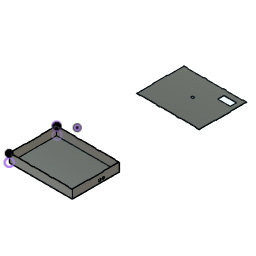
Final Submission (Autodesk Fusion 360 design; units mm, degrees)
Autodesk Fusion 360 part; units mm, degrees
sketch "Sketch1" plane through (0, 0, 0) normal (0, 0, 1) x (1, 0, 0)
  line L0 (-21.9872, 0) -> (-21.9872, 50)
  line L1 (-21.9872, 50) -> (-24.9872, 50)
  line L2 (-21.9872, 50) -> (-21.9872, 40)
  line L3 (-21.9872, 40) -> (-24.9872, 40)
  line L4 (-22, 40) -> (-22, 10)
  line L5 (-22, 10) -> (-25, 10)
  measures "d58" distance of L0.end
box "BoxPrimitive1" add length 300 width 450 height 50 placed x (0, 1, 0) y (-1, 0, 0) z (0, 0, 1) at (450, 0, 0) makes body 1
delete_face "DeleteFace1" 6 faces at (150, 100, 50) (0, 200, 16.6667) (300, 300, 16.6667) (450, 200, 16.6667) (300, 0, 16.6667) (150, 100, 0) on bodies 1
sketch "Sketch2" plane through (0, 0, 0) normal (0, 0, 1) x (1, 0, 0)
sketch "Sketch3" plane through (0, 0, 0) normal (0, 0, 1) x (1, 0, 0)
sketch "Sketch4" plane through (0, 0, 0) normal (0, 0, 1) x (1, 0, 0)
  line L0 (0, 0) -> (400, 0)
  line L1 (400, 0) -> (400, 3)
  line L2 (400, 3) -> (0, 3)
  line L3 (0, 3) -> (0, 0)
  dimension "d8" = 400
  constraint horizontal L0
  constraint vertical L1
  constraint horizontal L2
  constraint vertical L3
  constraint coincident L0.start L3.end
  measures "d8" distance of L0.start L0.end
extrude "Extrude1" add sketch "Sketch4" along normal blind 50 separate body makes body 2
sketch "Sketch5" plane through (0, 0, 0) normal (-1, 0, 0) x (0, -1, 0)
  line L0 (-3, 0) -> (0, 0)
  line L1 (0, 0) -> (0, 50)
  line L2 (0, 50) -> (-3, 50)
  line L3 (-3, 50) -> (-3, 0)
  line L4 (-3, 50) -> (0, 50)
  line L5 (0, 50) -> (0, 40)
  line L6 (0, 40) -> (-3, 40)
  line L7 (-3, 40) -> (-3, 50)
  dimension "d11" = 10
  constraint horizontal L4
  constraint vertical L5
  constraint horizontal L6
  constraint vertical L7
  constraint coincident L2.end L3.start
  measures "d11" distance of L2.end L6.end
sketch "Sketch6" plane through (0, 0, 0) normal (-1, 0, 0) x (0, -1, 0)
extrude "Extrude2" cut sketch "Sketch5" against normal blind 3 contours L1 L2 L3 L4 L5 L6 L7 bodies 2
sketch "Sketch7" plane through (0, 0, 0) normal (-1, 0, 0) x (0, -1, 0)
  line L0 (0, 40) -> (-3, 40)
  line L1 (-3, 40) -> (-3, 0)
  line L2 (-3, 0) -> (0, 0)
  line L3 (0, 0) -> (0, 40)
  line L4 (-3, 10) -> (0, 10)
  line L5 (0, 10) -> (0, 0)
  line L6 (0, 0) -> (-3, 0)
  line L7 (-3, 0) -> (-3, 10)
  constraint horizontal L4
  constraint vertical L5
  constraint horizontal L6
  constraint vertical L7
  constraint coincident L2.end L3.start
  constraint coincident L1 L4.start
extrude "Extrude3" cut sketch "Sketch7" against normal blind 3 contours L1 L2 L3 L4 L5 L6 L7 bodies 2
sketch "Sketch8" plane through (400, 0, 0) normal (1, 0, 0) x (0, 1, 0)
  line L0 (0, 0) -> (3, 0)
  line L1 (3, 0) -> (3, 50)
  line L2 (3, 50) -> (0, 50)
  line L3 (0, 50) -> (0, 0)
  line L4 (0, 50) -> (3.2755, 50)
  line L5 (3.2755, 50) -> (3.2755, 40)
  line L6 (3.2755, 40) -> (0, 40)
  line L7 (0, 40) -> (0, 50)
  line L8 (0, 40) -> (3, 40)
  line L9 (3, 40) -> (3, 10)
  line L10 (3, 10) -> (0, 10)
  line L11 (0, 10) -> (0, 40)
  line L12 (0, 10) -> (3, 10)
  line L13 (3, 10) -> (3, 0)
  line L14 (3, 0) -> (0, 0)
  line L15 (0, 0) -> (0, 10)
  dimension "d17" = 10
  dimension "d18" = 30
  constraint horizontal L4
  constraint vertical L5
  constraint horizontal L6
  constraint vertical L7
  constraint coincident L2.end L3.start
  constraint horizontal L8
  constraint vertical L9
  constraint horizontal L10
  constraint vertical L11
  constraint horizontal L12
  constraint vertical L13
  constraint horizontal L14
  constraint vertical L15
  constraint coincident L0.end L1.start
  measures "d17" distance of L2.end L6.end
  measures "d18" distance of L6.end L10.end
extrude "Extrude4" cut sketch "Sketch8" against normal blind 3 contours L1 L2 L3 L4 L6 L7 L8 bodies 2
sketch "Sketch9" plane through (0, 0, 0) normal (-1, 0, 0) x (0, -1, 0)
sketch "Sketch10" plane through (400, 0, 0) normal (1, 0, 0) x (0, 1, 0)
  line L0 (3, 40) -> (0, 40)
  line L1 (0, 40) -> (0, 0)
  line L2 (0, 0) -> (3, 0)
  line L3 (3, 0) -> (3, 40)
  line L4 (0, 0) -> (3, 0)
  line L5 (3, 0) -> (3, 10)
  line L6 (3, 10) -> (0, 10)
  line L7 (0, 10) -> (0, 0)
  dimension "d23" = 10
  constraint horizontal L4
  constraint vertical L5
  constraint horizontal L6
  constraint vertical L7
  constraint coincident L1.end L2.start
  measures "d23" distance of L1.end L6.end
extrude "Extrude5" cut sketch "Sketch10" against normal blind 3 contours L1 L2 L3 L4 L5 L6 L7 bodies 2
sketch "Sketch13" plane through (0, 0, 0) normal (0, 0, -1) x (1, 0, 0)
sketch "Sketch14" plane through (0, 0, 0) normal (0, 0, -1) x (1, 0, 0)
  line L0 (397, -3) -> (397, 0)
  line L1 (397, 0) -> (3, 0)
  line L2 (3, 0) -> (3, -3)
  line L3 (3, -3) -> (397, -3)
  line L4 (26.5, 0) -> (126.5, 0)
  line L5 (126.5, 0) -> (126.5, -2.9142)
  line L6 (126.5, -2.9142) -> (26.5, -2.9142)
  line L7 (26.5, -2.9142) -> (26.5, 0)
  dimension "d30" = 100
  constraint horizontal L4
  constraint vertical L5
  constraint horizontal L6
  constraint vertical L7
  constraint coincident L1 L4.start
  measures "d30" distance of L4.start L4.end
extrude "Extrude6" add sketch "Sketch14" along normal blind 3 contours L1 L4 L5 L6 L7 bodies 2
sketch "Sketch15" plane through (0, 0, 0) normal (0, 0, -1) x (1, 0, 0)
sketch "Sketch16" plane through (0, 0, 0) normal (0, 0, -1) x (1, 0, 0)
sketch "Sketch17" plane through (0, 0, 0) normal (0, 0, -1) x (1, 0, 0)
  line L0 (150, 0) -> (250, 0)
  line L1 (250, 0) -> (250, -3.0762)
  line L2 (250, -3.0762) -> (150, -3.0762)
  line L3 (150, -3.0762) -> (150, 0)
  dimension "d35" = 100
  constraint horizontal L0
  constraint vertical L1
  constraint horizontal L2
  constraint vertical L3
  measures "d35" distance of L0.start L0.end
sketch "Sketch18" plane through (0, 0, 0) normal (0, 0, -1) x (1, 0, 0)
extrude "Extrude7" add sketch "Sketch17" along normal blind 3 bodies 2
sketch "Sketch19" plane through (0, 0, 0) normal (0, 0, -1) x (1, 0, 0)
sketch "Sketch20" plane through (0, 0, 0) normal (0, 0, -1) x (1, 0, 0)
sketch "Sketch21" plane through (0, 0, 0) normal (0, 0, -1) x (1, 0, 0)
  line L0 (273.5, 0) -> (373.5, 0)
  line L1 (373.5, 0) -> (373.5, -3)
  line L2 (373.5, -3) -> (273.5, -3)
  line L3 (273.5, -3) -> (273.5, 0)
  dimension "d43" = 100
  constraint horizontal L0
  constraint vertical L1
  constraint horizontal L2
  constraint vertical L3
  measures "d43" distance of L0.start L0.end
extrude "Extrude8" add sketch "Sketch21" along normal blind 3 bodies 2
sketch "Sketch23" plane through (0, 0, 0) normal (0, 0, 1) x (1, 0, 0)
sketch "Sketch24" plane through (0, 0, 0) normal (0, 0, 1) x (1, 0, 0)
  line L0 (0, -2) -> (3, -2)
  line L1 (3, -2) -> (3, -302)
  line L2 (3, -302) -> (0, -302)
  line L3 (0, -302) -> (0, -2)
  dimension "d47" = 3
  dimension "d48" = 300
  constraint horizontal L0
  constraint vertical L1
  constraint horizontal L2
  constraint vertical L3
  measures "d47" distance of L0.start L0.end
  measures "d48" distance of L0.start L2.end
sketch "Sketch22" plane through (0, 0, 0) normal (0, -1, 0) x (1, 0, 0)
extrude "Extrude9" add sketch "Sketch24" along normal blind 50 separate body makes body 3
move_body "MoveFace1" bodies 3 to x (1, 0, 0) y (0, 1, 0) z (0, 0, 1) at (-24.9872, -104.133, 0) on bodies 3
sketch "Sketch55" plane through (0, 0, 3) normal (0, 0, 1) x (-1, 0, 0)
  line L0 (-192.7778, -526.1003) -> (-207.7778, -526.1003)
  line L1 (-207.7778, -526.1003) -> (-207.7778, -514.1003)
  line L2 (-207.7778, -514.1003) -> (-192.7778, -514.1003)
  line L3 (-192.7778, -514.1003) -> (-192.7778, -526.1003)
  dimension "d161" = 15
  dimension "d162" = 12
  constraint horizontal L0
  constraint vertical L1
  constraint horizontal L2
  constraint vertical L3
  measures "d161" distance of L0.start L0.end
  measures "d162" distance of L0.start L2.end
sketch "Sketch25" plane through (0, -106.133, 0) normal (0, 1, 0) x (-1, 0, 0)
  line L0 (24.9872, 50) -> (21.9872, 50)
  line L1 (21.9872, 50) -> (24.9872, 50)
  line L2 (21.9872, 40) -> (21.9872, 50)
  dimension "d51" = 10
  constraint horizontal L1
  constraint vertical L2
  constraint coincident L0.end L1.start
  measures "d51" distance of L0.end L2.start
sketch "Sketch56" plane through (0, 0, 3) normal (0, 0, 1) x (1, 0, 0)
sketch "Sketch26" plane through (0, -106.133, 0) normal (0, 1, 0) x (-1, 0, 0)
sketch "Sketch27" plane through (0, -106.133, 0) normal (0, 1, 0) x (-1, 0, 0)
  line L0 (22, 40) -> (25.1085, 40)
  line L1 (25.1085, 40) -> (25.1085, 10)
  line L2 (25.1085, 10) -> (22, 10)
  line L3 (22, 10) -> (22, 40)
  dimension "d54" = 30
  constraint horizontal L0
  constraint vertical L1
  constraint horizontal L2
  constraint vertical L3
  measures "d54" distance of L0.start L2.end
sketch "Sketch28" plane through (0, -106.133, 0) normal (0, 1, 0) x (-1, 0, 0)
extrude "Extrude10" cut sketch "Sketch27" against normal blind 3 bodies 3
delete_face "DeleteFace2" 1 faces at (-22, -108.133, 20) on bodies 3
sketch "Sketch29" plane through (0, -406.133, 0) normal (0, -1, 0) x (1, 0, 0)
  line L0 (-24.9872, 0) -> (-21.9872, 0)
  line L1 (-21.9872, 0) -> (-21.9872, 50)
  line L2 (-21.9872, 50) -> (-24.9872, 50)
  line L3 (-24.9872, 50) -> (-21.9872, 50)
  line L4 (-21.9872, 50) -> (-21.9872, 40)
  line L5 (-21.9872, 40) -> (-24.9872, 40)
  line L6 (-24.9872, 40) -> (-24.9872, 50)
  dimension "d57" = 10
  dimension "d58" = 3
  constraint horizontal L3
  constraint vertical L4
  constraint horizontal L5
  constraint vertical L6
  constraint coincident L2.end L3.start
  measures "d57" distance of L2.end L5.end
  measures "d58" distance of L2.end L1.end
sketch "Sketch30" plane through (0, -406.133, 0) normal (0, -1, 0) x (1, 0, 0)
sketch "Sketch31" plane through (-23.4872, -406.133, 20) normal (0, -1, 0) x (1, 0, 0)
sketch "Sketch32" plane through (-23.4872, -406.133, 20) normal (0, -1, 0) x (1, 0, 0)
sketch "Sketch33" plane through (0, -406.133, 0) normal (0, -1, 0) x (1, 0, 0)
  line L0 (-25, 40) -> (-22, 40)
  line L1 (-22, 40) -> (-22, 10)
  line L2 (-22, 10) -> (-25, 10)
  line L3 (-25, 10) -> (-25, 40)
  constraint horizontal L0
  constraint vertical L1
  constraint horizontal L2
  constraint vertical L3
extrude "Extrude11" cut sketch "Sketch33" against normal blind 3 bodies 3
delete_face "DeleteFace3" 1 faces at (-22, -405.133, 30) on bodies 3
sketch "Sketch34" plane through (0, 0, 0) normal (0, 0, -1) x (1, 0, 0)
  line L0 (-21.9872, 406.133) -> (-24.9872, 406.133)
  line L1 (-21.9872, 106.133) -> (-21.9872, 406.133)
sketch "Sketch35" plane through (0, 0, 0) normal (0, 0, -1) x (1, 0, 0)
  line L0 (-25, 109) -> (-22, 109)
  line L1 (-22, 109) -> (-22, 209)
  line L2 (-22, 209) -> (-25, 209)
  line L3 (-25, 209) -> (-25, 109)
  dimension "d65" = 100
  constraint horizontal L0
  constraint vertical L1
  constraint horizontal L2
  constraint vertical L3
  measures "d65" distance of L0.start L2.end
extrude "Extrude12" add sketch "Sketch35" along normal blind 3 bodies 3
sketch "Sketch36" plane through (0, 0, 0) normal (0, 0, -1) x (1, 0, 0)
sketch "Sketch37" plane through (0, 0, 0) normal (0, 0, -1) x (1, 0, 0)
  line L0 (-25, 403) -> (-22, 403)
  line L1 (-22, 403) -> (-22, 303)
  line L2 (-22, 303) -> (-25, 303)
  line L3 (-25, 303) -> (-25, 403)
  dimension "d69" = 100
  constraint horizontal L0
  constraint vertical L1
  constraint horizontal L2
  constraint vertical L3
  measures "d69" distance of L0.start L2.end
extrude "Extrude13" add sketch "Sketch37" along normal blind 3 bodies 3
copy_body "CopyPasteBodies1" bodies 3 makes body 4
move_body "Move1" bodies 4 to x (1, 0, 0) y (0, 1, 0) z (0, 0, 1) at (550, 0, 0)
copy_body "CopyPasteBodies2" bodies 2 makes body 5
move_body "Move2" bodies 5 to x (1, 0, 0) y (0, 1, 0) z (0, 0, 1) at (0, -430, 0)
move_body "Align1" bodies 5 to x (1, 0, 0) y (0, 1, 0) z (0, 0, 1) at (-24.9872, 23.867, 0)
move_body "Align2" bodies 2 to x (1, 0, 0) y (0, 1, 0) z (0, 0, 1) at (-24.9872, -109.133, 0)
move_body "Align3" bodies 4 to x (1, 0, 0) y (0, 1, 0) z (0, 0, 1) at (-153, 0, 0)
hole "Hole1" at (375.0128, -209.5503, 16.3577) direction (-1, 0, 0) diameter 15 depth 18 tip angle 118 bodies 4
sketch "Sketch38" plane through (0, -406.133, 0) normal (0, -1, 0) x (1, 0, 0)
sketch "Sketch39" plane through (0, 0, 0) normal (0, 0, 1) x (1, 0, 0)
  line L0 (0, 0) -> (400, 0)
  line L1 (400, 0) -> (400, 300)
  line L2 (400, 300) -> (0, 300)
  line L3 (0, 300) -> (0, 0)
  dimension "d75" = 300
  dimension "d76" = 400
  constraint horizontal L0
  constraint vertical L1
  constraint horizontal L2
  constraint vertical L3
  constraint coincident L0.start L3.end
  measures "d75" distance of L0.start L2.end
  measures "d76" distance of L0.start L0.end
sketch "Sketch40" plane through (0, 0, 0) normal (0, 0, 1) x (1, 0, 0)
  line L0 (0, 0) -> (26.5, 0)
  line L1 (26.5, 0) -> (26.5, 3)
  line L2 (26.5, 3) -> (0, 3)
  line L3 (0, 3) -> (0, 0)
  line L4 (26.5, 3) -> (126.5, 3)
  line L5 (126.5, 3) -> (126.5, 0)
  line L6 (126.5, 0) -> (26.5, 0)
  line L7 (26.5, 0) -> (26.5, 3)
  line L8 (126.5, 3) -> (150, 3)
  line L9 (150, 3) -> (150, 0)
  line L10 (150, 0) -> (126.5, 0)
  line L11 (126.5, 0) -> (126.5, 3)
  line L12 (150, 3) -> (250, 3)
  line L13 (250, 3) -> (250, 0)
  line L14 (250, 0) -> (150, 0)
  line L15 (150, 0) -> (150, 3)
  line L16 (250, 3) -> (273.5, 3)
  line L17 (273.5, 3) -> (273.5, 0)
  line L18 (273.5, 0) -> (250, 0)
  line L19 (250, 0) -> (250, 3)
  line L20 (273.5, 3) -> (373.5, 3)
  line L21 (373.5, 3) -> (373.5, 0)
  line L22 (373.5, 0) -> (273.5, 0)
  line L23 (273.5, 0) -> (273.5, 3)
  line L24 (373.5, 3) -> (400, 3)
  line L25 (400, 3) -> (400, 0)
  line L26 (400, 0) -> (373.5, 0)
  line L27 (373.5, 0) -> (373.5, 3)
  dimension "d77" = 26.5
  dimension "d78" = 3
  dimension "d79" = 100
  dimension "d80" = 3
  dimension "d81" = 23.5
  dimension "d82" = 3
  dimension "d83" = 100
  dimension "d84" = 3
  dimension "d85" = 23.5
  dimension "d86" = 3
  dimension "d87" = 100
  constraint horizontal L0
  constraint vertical L1
  constraint horizontal L2
  constraint vertical L3
  constraint coincident L0.start L3.end
  constraint horizontal L4
  constraint vertical L5
  constraint horizontal L6
  constraint vertical L7
  constraint horizontal L8
  constraint vertical L9
  constraint horizontal L10
  constraint vertical L11
  constraint horizontal L12
  constraint vertical L13
  constraint horizontal L14
  constraint vertical L15
  constraint horizontal L16
  constraint vertical L17
  constraint horizontal L18
  constraint vertical L19
  constraint horizontal L20
  constraint vertical L21
  constraint horizontal L22
  constraint vertical L23
  constraint horizontal L24
  constraint vertical L25
  constraint horizontal L26
  constraint vertical L27
  measures "d77" distance of L0.start L0.end
  measures "d78" distance of L0.start L2.end
  measures "d79" distance of L1.end L4.end
  measures "d80" distance of L1.end L0.end
  measures "d81" distance of L4.end L8.end
  measures "d82" distance of L4.end L5.end
  measures "d83" distance of L8.end L12.end
  measures "d84" distance of L8.end L9.end
  measures "d85" distance of L12.end L16.end
  measures "d86" distance of L12.end L13.end
  measures "d87" distance of L16.end L20.end
sketch "Sketch41" plane through (0, 0, 0) normal (0, 0, 1) x (1, 0, 0)
  line L0 (0, 3) -> (3, 3)
  line L1 (3, 3) -> (3, 103)
  line L2 (3, 103) -> (0, 103)
  line L3 (0, 103) -> (0, 3)
  line L4 (3, 103) -> (0, 103)
  line L5 (0, 103) -> (0, 197)
  line L6 (0, 197) -> (3, 197)
  line L7 (3, 197) -> (3, 103)
  line L8 (3, 197) -> (0, 197)
  line L9 (0, 197) -> (0, 297)
  line L10 (0, 297) -> (3, 297)
  line L11 (3, 297) -> (3, 197)
  dimension "d88" = 100
  dimension "d89" = 3
  dimension "d90" = 3
  dimension "d91" = 94
  dimension "d92" = 3
  dimension "d93" = 100
  constraint horizontal L0
  constraint vertical L1
  constraint horizontal L2
  constraint vertical L3
  constraint horizontal L4
  constraint vertical L5
  constraint horizontal L6
  constraint vertical L7
  constraint horizontal L8
  constraint vertical L9
  constraint horizontal L10
  constraint vertical L11
  measures "d88" distance of L0.start L2.end
  measures "d89" distance of L0.start L0.end
  measures "d90" distance of L1.end L2.end
  measures "d91" distance of L1.end L6.end
  measures "d92" distance of L6.end L5.end
  measures "d93" distance of L6.end L10.end
sketch "Sketch42" plane through (0, 0, 0) normal (0, 0, 1) x (1, 0, 0)
  line L0 (400, 3) -> (397, 3)
  line L1 (397, 3) -> (397, 103)
  line L2 (397, 103) -> (400, 103)
  line L3 (400, 103) -> (400, 3)
  line L4 (397, 103) -> (400, 103)
  line L5 (400, 103) -> (400, 197)
  line L6 (400, 197) -> (397, 197)
  line L7 (397, 197) -> (397, 103)
  line L8 (397, 197) -> (400, 197)
  line L9 (400, 197) -> (400, 297)
  line L10 (400, 297) -> (397, 297)
  line L11 (397, 297) -> (397, 197)
  dimension "d94" = 100
  dimension "d95" = 94
  dimension "d96" = 100
  constraint horizontal L0
  constraint vertical L1
  constraint horizontal L2
  constraint vertical L3
  constraint horizontal L4
  constraint vertical L5
  constraint horizontal L6
  constraint vertical L7
  constraint horizontal L8
  constraint vertical L9
  constraint horizontal L10
  constraint vertical L11
  measures "d94" distance of L0.start L2.end
  measures "d95" distance of L1.end L6.end
  measures "d96" distance of L6.end L10.end
sketch "Sketch43" plane through (0, 0, 0) normal (0, 0, 1) x (1, 0, 0)
  line L0 (400, 297) -> (373.5, 297)
  line L1 (373.5, 297) -> (373.5, 300)
  line L2 (373.5, 300) -> (400, 300)
  line L3 (400, 300) -> (400, 297)
  line L4 (373.5, 297) -> (273.5, 297)
  line L5 (273.5, 297) -> (273.5, 300)
  line L6 (273.5, 300) -> (373.5, 300)
  line L7 (373.5, 300) -> (373.5, 297)
  line L8 (273.5, 297) -> (250, 297)
  line L9 (250, 297) -> (250, 300)
  line L10 (250, 300) -> (273.5, 300)
  line L11 (273.5, 300) -> (273.5, 297)
  line L12 (250, 297) -> (150, 297)
  line L13 (150, 297) -> (150, 300)
  line L14 (150, 300) -> (250, 300)
  line L15 (250, 300) -> (250, 297)
  line L16 (150, 297) -> (126.5, 297)
  line L17 (126.5, 297) -> (126.5, 300)
  line L18 (126.5, 300) -> (150, 300)
  line L19 (150, 300) -> (150, 297)
  line L20 (126.5, 297) -> (26.5, 297)
  line L21 (26.5, 297) -> (26.5, 300)
  line L22 (26.5, 300) -> (126.5, 300)
  line L23 (126.5, 300) -> (126.5, 297)
  line L24 (26.5, 297) -> (0, 297)
  line L25 (0, 297) -> (0, 300)
  line L26 (0, 300) -> (26.5, 300)
  line L27 (26.5, 300) -> (26.5, 297)
  dimension "d97" = 26.5
  dimension "d98" = 100
  dimension "d99" = 23.5
  dimension "d100" = 100
  dimension "d101" = 23.5
  dimension "d102" = 100
  constraint horizontal L0
  constraint vertical L1
  constraint horizontal L2
  constraint vertical L3
  constraint horizontal L4
  constraint vertical L5
  constraint horizontal L6
  constraint vertical L7
  constraint horizontal L8
  constraint vertical L9
  constraint horizontal L10
  constraint vertical L11
  constraint horizontal L12
  constraint vertical L13
  constraint horizontal L14
  constraint vertical L15
  constraint horizontal L16
  constraint vertical L17
  constraint horizontal L18
  constraint vertical L19
  constraint horizontal L20
  constraint vertical L21
  constraint horizontal L22
  constraint vertical L23
  constraint horizontal L24
  constraint vertical L25
  constraint horizontal L26
  constraint vertical L27
  measures "d97" distance of L0.start L0.end
  measures "d98" distance of L0.end L4.end
  measures "d99" distance of L4.end L8.end
  measures "d100" distance of L8.end L12.end
  measures "d101" distance of L12.end L16.end
  measures "d102" distance of L16.end L20.end
extrude "Extrude14" add sketch "Sketch39" along normal blind 3 separate body makes body 6
extrude "Extrude15" cut sketch "Sketch41" along normal blind 3 contours L0 L1 L2 L3 L4 bodies 6
extrude "Extrude16" cut sketch "Sketch40" along normal blind 3 contours L1 L4 L5 L6 L7 L11 | L9 L12 L13 L14 L15 L19 | L17 L20 L21 L22 L23 L27 bodies 6
extrude "Extrude17" cut sketch "Sketch42" along normal blind 3 contours L0 L1 L2 L3 L4 | L6 L8 L9 L10 L11 bodies 6
extrude "Extrude18" cut sketch "Sketch43" along normal blind 3 contours L1 L4 L5 L6 L7 L11 | L9 L12 L13 L14 L15 L19 | L17 L20 L21 L22 L23 L27 bodies 6
sketch "Sketch44" plane through (0, 0, 3) normal (0, 0, 1) x (-1, 0, 0)
  line L0 (-273.5, -297) -> (-273.5, -300)
  line L1 (-273.5, -300) -> (-250, -300)
  line L2 (-250, -300) -> (-250, -297)
  line L3 (-250, -297) -> (-150, -297)
  line L4 (-150, -297) -> (-150, -300)
  line L5 (-150, -300) -> (-126.5, -300)
  line L6 (-126.5, -300) -> (-126.5, -297)
  line L7 (-126.5, -297) -> (-26.5, -297)
  line L8 (-26.5, -297) -> (-26.5, -300)
  line L9 (-26.5, -300) -> (0, -300)
  line L10 (0, -300) -> (0, -103)
  line L11 (0, -103) -> (-3, -103)
  line L12 (-3, -103) -> (-3, -3)
  line L13 (-3, -3) -> (0, -3)
  line L14 (0, -3) -> (0, 0)
  line L15 (0, 0) -> (-26.5, 0)
  line L16 (-26.5, 0) -> (-26.5, -3)
  line L17 (-26.5, -3) -> (-126.5, -3)
  line L18 (-126.5, -3) -> (-126.5, 0)
  line L19 (-126.5, 0) -> (-150, 0)
  line L20 (-150, 0) -> (-150, -3)
  line L21 (-150, -3) -> (-250, -3)
  line L22 (-250, -3) -> (-250, 0)
  line L23 (-250, 0) -> (-273.5, 0)
  line L24 (-273.5, 0) -> (-273.5, -3)
  line L25 (-273.5, -3) -> (-373.5, -3)
  line L26 (-373.5, -3) -> (-373.5, 0)
  line L27 (-373.5, 0) -> (-400, 0)
  line L28 (-400, 0) -> (-400, -3)
  line L29 (-400, -3) -> (-397, -3)
  line L30 (-397, -3) -> (-397, -103)
  line L31 (-397, -103) -> (-400, -103)
  line L32 (-400, -103) -> (-400, -197)
  line L33 (-400, -197) -> (-397, -197)
  line L34 (-397, -197) -> (-397, -297)
  line L35 (-397, -297) -> (-400, -297)
  line L36 (-400, -297) -> (-400, -300)
  line L37 (-400, -300) -> (-373.5, -300)
  line L38 (-373.5, -300) -> (-373.5, -297)
  line L39 (-373.5, -297) -> (-273.5, -297)
  line L40 (0, -300) -> (-3, -300)
  line L41 (-3, -300) -> (-3, -297)
  line L42 (-3, -297) -> (0, -297)
  line L43 (0, -297) -> (0, -300)
  line L44 (0, -297) -> (-3, -297)
  line L45 (-3, -297) -> (-3, -197)
  line L46 (-3, -197) -> (0, -197)
  line L47 (0, -197) -> (0, -297)
  dimension "d113" = 3
  dimension "d114" = 3
  dimension "d115" = 100
  dimension "d116" = 3
  constraint horizontal L40
  constraint vertical L41
  constraint horizontal L42
  constraint vertical L43
  constraint coincident L9.end L10.start
  constraint horizontal L44
  constraint vertical L45
  constraint horizontal L46
  constraint vertical L47
  measures "d113" distance of L9.end L42.end
  measures "d114" distance of L9.end L40.end
  measures "d115" distance of L42.end L46.end
  measures "d116" distance of L42.end L41.end
extrude "Extrude19" cut sketch "Sketch44" against normal blind 3 contours L10 L42 L44 L45 L46 L47 bodies 6
copy_body "CopyPasteBodies3" bodies 6 makes body 7
move_body "Move3" bodies 7 to x (1, 0, 0) y (0, 1, 0) z (0, 0, 1) at (0, 375, 0)
move_body "Align4" bodies 6 to x (1, 0, 0) y (0, 1, 0) z (0, 0, 1) at (-25, -406, -3)
sketch "Sketch45" plane through (0, 0, 50) normal (0, 0, 1) x (-1, 0, 0)
  line L0 (24.9872, 406.133) -> (21.9872, 406.133)
  line L1 (21.9872, 406.133) -> (21.9872, 106.133)
  line L2 (21.9872, 106.133) -> (24.9872, 106.133)
  line L3 (24.9872, 106.133) -> (24.9872, 406.133)
  line L4 (24.9872, 106.133) -> (21.9872, 106.133)
  line L5 (21.9872, 106.133) -> (21.9872, 109.133)
  line L6 (21.9872, 109.133) -> (24.9872, 109.133)
  line L7 (24.9872, 109.133) -> (24.9872, 106.133)
  line L8 (24.9872, 109.133) -> (21.9872, 109.133)
  line L9 (21.9872, 109.133) -> (21.9872, 209.133)
  line L10 (21.9872, 209.133) -> (24.9872, 209.133)
  line L11 (24.9872, 209.133) -> (24.9872, 109.133)
  line L12 (24.9872, 209.133) -> (21.9872, 209.133)
  line L13 (21.9872, 209.133) -> (21.9872, 303.133)
  line L14 (21.9872, 303.133) -> (24.9872, 303.133)
  line L15 (24.9872, 303.133) -> (24.9872, 209.133)
  line L16 (24.9872, 303.133) -> (21.9872, 303.133)
  line L17 (21.9872, 303.133) -> (21.9872, 403.133)
  line L18 (21.9872, 403.133) -> (24.9872, 403.133)
  line L19 (24.9872, 403.133) -> (24.9872, 303.133)
  dimension "d119" = 3
  dimension "d120" = 100
  dimension "d121" = 94
  dimension "d122" = 3
  dimension "d123" = 100
  dimension "d124" = 3
  constraint horizontal L4
  constraint vertical L5
  constraint horizontal L6
  constraint vertical L7
  constraint coincident L2.end L3.start
  constraint horizontal L8
  constraint vertical L9
  constraint horizontal L10
  constraint vertical L11
  constraint horizontal L12
  constraint vertical L13
  constraint horizontal L14
  constraint vertical L15
  constraint horizontal L16
  constraint vertical L17
  constraint horizontal L18
  constraint vertical L19
  measures "d119" distance of L2.end L6.end
  measures "d120" distance of L6.end L10.end
  measures "d121" distance of L10.end L14.end
  measures "d122" distance of L10.end L9.end
  measures "d123" distance of L14.end L18.end
  measures "d124" distance of L14.end L13.end
extrude "Extrude20" add sketch "Sketch45" along normal blind 3 contours L1 L3 L14 L16 L17 L18 L19 | L1 L3 L6 L8 L9 L10 L11 L12 bodies 3 4 6 2 5
sketch "Sketch46" plane through (0, 0, 50) normal (0, 0, 1) x (-1, 0, 0)
  line L0 (24.9872, 109.133) -> (21.9872, 109.133)
  line L1 (21.9872, 109.133) -> (-372.0128, 109.133)
  line L2 (-372.0128, 109.133) -> (-372.0128, 106.133)
  line L3 (-372.0128, 106.133) -> (24.9872, 106.133)
  line L4 (24.9872, 106.133) -> (24.9872, 109.133)
  line L5 (24.9872, 106.133) -> (-1.5128, 106.133)
  line L6 (-1.5128, 106.133) -> (-1.5128, 109.133)
  line L7 (-1.5128, 109.133) -> (24.9872, 109.133)
  line L8 (24.9872, 109.133) -> (24.9872, 106.133)
  line L9 (-1.5128, 106.133) -> (-101.5128, 106.133)
  line L10 (-101.5128, 106.133) -> (-101.5128, 109.133)
  line L11 (-101.5128, 109.133) -> (-1.5128, 109.133)
  line L12 (-1.5128, 109.133) -> (-1.5128, 106.133)
  line L13 (-101.5128, 106.133) -> (-125.0128, 106.133)
  line L14 (-125.0128, 106.133) -> (-125.0128, 109.133)
  line L15 (-125.0128, 109.133) -> (-101.5128, 109.133)
  line L16 (-101.5128, 109.133) -> (-101.5128, 106.133)
  line L17 (-125.0128, 106.133) -> (-225.0128, 106.133)
  line L18 (-225.0128, 106.133) -> (-225.0128, 109.133)
  line L19 (-225.0128, 109.133) -> (-125.0128, 109.133)
  line L20 (-125.0128, 109.133) -> (-125.0128, 106.133)
  line L21 (-225.0128, 106.133) -> (-248.5128, 106.133)
  line L22 (-248.5128, 106.133) -> (-248.5128, 109.133)
  line L23 (-248.5128, 109.133) -> (-225.0128, 109.133)
  line L24 (-225.0128, 109.133) -> (-225.0128, 106.133)
  line L25 (-248.5128, 106.133) -> (-348.5128, 106.133)
  line L26 (-348.5128, 106.133) -> (-348.5128, 109.133)
  line L27 (-348.5128, 109.133) -> (-248.5128, 109.133)
  line L28 (-248.5128, 109.133) -> (-248.5128, 106.133)
  dimension "d127" = 26.5
  dimension "d128" = 3
  dimension "d129" = 100
  dimension "d130" = 23.5
  dimension "d131" = 100
  dimension "d132" = 23.5
  dimension "d133" = 100
  constraint horizontal L5
  constraint vertical L6
  constraint horizontal L7
  constraint vertical L8
  constraint coincident L3.end L4.start
  constraint horizontal L9
  constraint vertical L10
  constraint horizontal L11
  constraint vertical L12
  constraint horizontal L13
  constraint vertical L14
  constraint horizontal L15
  constraint vertical L16
  constraint horizontal L17
  constraint vertical L18
  constraint horizontal L19
  constraint vertical L20
  constraint horizontal L21
  constraint vertical L22
  constraint horizontal L23
  constraint vertical L24
  constraint horizontal L25
  constraint vertical L26
  constraint horizontal L27
  constraint vertical L28
  measures "d127" distance of L3.end L5.end
  measures "d128" distance of L3.end L0.start
  measures "d129" distance of L5.end L9.end
  measures "d130" distance of L9.end L13.end
  measures "d131" distance of L13.end L17.end
  measures "d132" distance of L17.end L21.end
  measures "d133" distance of L21.end L25.end
extrude "Extrude21" add sketch "Sketch46" along normal blind 3 contours L1 L3 L6 L9 L10 L11 L12 L16 | L1 L3 L14 L17 L18 L19 L20 L24 | L1 L3 L22 L25 L26 L27 L28 bodies 3
sketch "Sketch47" plane through (0, 0, 50) normal (0, 0, 1) x (-1, 0, 0)
  line L0 (-372.0128, 406.133) -> (-375.0128, 406.133)
  line L1 (-375.0128, 406.133) -> (-375.0128, 106.133)
  line L2 (-375.0128, 106.133) -> (-372.0128, 106.133)
  line L3 (-372.0128, 106.133) -> (-372.0128, 406.133)
  line L4 (-372.0128, 106.133) -> (-375.0128, 106.133)
  line L5 (-375.0128, 106.133) -> (-375.0128, 109.133)
  line L6 (-375.0128, 109.133) -> (-372.0128, 109.133)
  line L7 (-372.0128, 109.133) -> (-372.0128, 106.133)
  line L8 (-372.0128, 109.133) -> (-375.0128, 109.133)
  line L9 (-375.0128, 109.133) -> (-375.0128, 209.133)
  line L10 (-375.0128, 209.133) -> (-372.0128, 209.133)
  line L11 (-372.0128, 209.133) -> (-372.0128, 109.133)
  line L12 (-372.0128, 209.133) -> (-375.0128, 209.133)
  line L13 (-375.0128, 209.133) -> (-375.0128, 303.133)
  line L14 (-375.0128, 303.133) -> (-372.0128, 303.133)
  line L15 (-372.0128, 303.133) -> (-372.0128, 209.133)
  line L16 (-372.0128, 303.133) -> (-375.0128, 303.133)
  line L17 (-375.0128, 303.133) -> (-375.0128, 403.133)
  line L18 (-375.0128, 403.133) -> (-372.0128, 403.133)
  line L19 (-372.0128, 403.133) -> (-372.0128, 303.133)
  dimension "d136" = 3
  dimension "d137" = 100
  dimension "d138" = 3
  dimension "d139" = 94
  dimension "d140" = 100
  constraint horizontal L4
  constraint vertical L5
  constraint horizontal L6
  constraint vertical L7
  constraint coincident L2.end L3.start
  constraint horizontal L8
  constraint vertical L9
  constraint horizontal L10
  constraint vertical L11
  constraint horizontal L12
  constraint vertical L13
  constraint horizontal L14
  constraint vertical L15
  constraint horizontal L16
  constraint vertical L17
  constraint horizontal L18
  constraint vertical L19
  measures "d136" distance of L2.end L6.end
  measures "d137" distance of L6.end L10.end
  measures "d138" distance of L6.end L5.end
  measures "d139" distance of L10.end L14.end
  measures "d140" distance of L14.end L18.end
extrude "Extrude22" add sketch "Sketch47" along normal blind 3 contours L1 L3 L14 L16 L17 L18 L19 | L1 L3 L6 L8 L9 L10 L11 L12 bodies 4 6 3
sketch "Sketch48" plane through (0, 0, 50) normal (0, 0, 1) x (-1, 0, 0)
  line L0 (-375.0128, 403.133) -> (-372.0128, 403.133)
  line L1 (-372.0128, 403.133) -> (21.9872, 403.133)
  line L2 (21.9872, 403.133) -> (24.9872, 403.133)
  line L3 (24.9872, 403.133) -> (24.9872, 406.133)
  line L4 (24.9872, 406.133) -> (-375.0128, 406.133)
  line L5 (-375.0128, 406.133) -> (-375.0128, 403.133)
  line L6 (-375.0128, 403.133) -> (-348.5128, 403.133)
  line L7 (-348.5128, 403.133) -> (-348.5128, 406.133)
  line L8 (-348.5128, 406.133) -> (-375.0128, 406.133)
  line L9 (-375.0128, 406.133) -> (-375.0128, 403.133)
  line L10 (-348.5128, 403.133) -> (-248.5128, 403.133)
  line L11 (-248.5128, 403.133) -> (-248.5128, 406.133)
  line L12 (-248.5128, 406.133) -> (-348.5128, 406.133)
  line L13 (-348.5128, 406.133) -> (-348.5128, 403.133)
  line L14 (-248.5128, 403.133) -> (-225.0128, 403.133)
  line L15 (-225.0128, 403.133) -> (-225.0128, 406.133)
  line L16 (-225.0128, 406.133) -> (-248.5128, 406.133)
  line L17 (-248.5128, 406.133) -> (-248.5128, 403.133)
  line L18 (-225.0128, 403.133) -> (-125.0128, 403.133)
  line L19 (-125.0128, 403.133) -> (-125.0128, 406.133)
  line L20 (-125.0128, 406.133) -> (-225.0128, 406.133)
  line L21 (-225.0128, 406.133) -> (-225.0128, 403.133)
  line L22 (-125.0128, 403.133) -> (-101.5128, 403.133)
  line L23 (-101.5128, 403.133) -> (-101.5128, 406.133)
  line L24 (-101.5128, 406.133) -> (-125.0128, 406.133)
  line L25 (-125.0128, 406.133) -> (-125.0128, 403.133)
  line L26 (-101.5128, 403.133) -> (-1.5128, 403.133)
  line L27 (-1.5128, 403.133) -> (-1.5128, 406.133)
  line L28 (-1.5128, 406.133) -> (-101.5128, 406.133)
  line L29 (-101.5128, 406.133) -> (-101.5128, 403.133)
  dimension "d143" = 26.5
  dimension "d144" = 100
  dimension "d145" = 23.5
  dimension "d146" = 100
  dimension "d147" = 23.5
  dimension "d148" = 100
  constraint horizontal L6
  constraint vertical L7
  constraint horizontal L8
  constraint vertical L9
  constraint coincident L0.start L5.end
  constraint horizontal L10
  constraint vertical L11
  constraint horizontal L12
  constraint vertical L13
  constraint horizontal L14
  constraint vertical L15
  constraint horizontal L16
  constraint vertical L17
  constraint horizontal L18
  constraint vertical L19
  constraint horizontal L20
  constraint vertical L21
  constraint horizontal L22
  constraint vertical L23
  constraint horizontal L24
  constraint vertical L25
  constraint horizontal L26
  constraint vertical L27
  constraint horizontal L28
  constraint vertical L29
  measures "d143" distance of L0.start L6.end
  measures "d144" distance of L6.end L10.end
  measures "d145" distance of L10.end L14.end
  measures "d146" distance of L14.end L18.end
  measures "d147" distance of L18.end L22.end
  measures "d148" distance of L22.end L26.end
extrude "Extrude23" add sketch "Sketch48" along normal blind 3 contours L1 L4 L7 L10 L11 L12 L13 L17 | L1 L4 L15 L18 L19 L20 L21 L25 | L1 L4 L23 L26 L27 L28 L29 bodies 4
move_body "Align5" bodies 4 to x (1, 0, 0) y (0, 1, 0) z (0, 0, 1) at (0, 0.133, 0)
sketch "Sketch49" plane through (0, 0, 3) normal (0, 0, 1) x (-1, 0, 0)
  line L0 (-3, -572) -> (0, -572)
  line L1 (0, -572) -> (0, -478)
  line L2 (0, -478) -> (-3, -478)
  line L3 (-3, -478) -> (-3, -378)
  line L4 (-3, -378) -> (0, -378)
  line L5 (0, -378) -> (0, -375)
  line L6 (0, -375) -> (-26.5, -375)
  line L7 (-26.5, -375) -> (-26.5, -378)
  line L8 (-26.5, -378) -> (-126.5, -378)
  line L9 (-126.5, -378) -> (-126.5, -375)
  line L10 (-126.5, -375) -> (-150, -375)
  line L11 (-150, -375) -> (-150, -378)
  line L12 (-150, -378) -> (-250, -378)
  line L13 (-250, -378) -> (-250, -375)
  line L14 (-250, -375) -> (-273.5, -375)
  line L15 (-273.5, -375) -> (-273.5, -378)
  line L16 (-273.5, -378) -> (-373.5, -378)
  line L17 (-373.5, -378) -> (-373.5, -375)
  line L18 (-373.5, -375) -> (-400, -375)
  line L19 (-400, -375) -> (-400, -378)
  line L20 (-400, -378) -> (-397, -378)
  line L21 (-397, -378) -> (-397, -478)
  line L22 (-397, -478) -> (-400, -478)
  line L23 (-400, -478) -> (-400, -572)
  line L24 (-400, -572) -> (-397, -572)
  line L25 (-397, -572) -> (-397, -672)
  line L26 (-397, -672) -> (-400, -672)
  line L27 (-400, -672) -> (-400, -675)
  line L28 (-400, -675) -> (-373.5, -675)
  line L29 (-373.5, -675) -> (-373.5, -672)
  line L30 (-373.5, -672) -> (-273.5, -672)
  line L31 (-273.5, -672) -> (-273.5, -675)
  line L32 (-273.5, -675) -> (-250, -675)
  line L33 (-250, -675) -> (-250, -672)
  line L34 (-250, -672) -> (-150, -672)
  line L35 (-150, -672) -> (-150, -675)
  line L36 (-150, -675) -> (-126.5, -675)
  line L37 (-126.5, -675) -> (-126.5, -672)
  line L38 (-126.5, -672) -> (-26.5, -672)
  line L39 (-26.5, -672) -> (-26.5, -675)
  line L40 (-26.5, -675) -> (0, -675)
  line L41 (0, -675) -> (0, -672)
  line L42 (0, -672) -> (-3, -672)
  line L43 (-3, -672) -> (-3, -572)
  line L44 (-370, -640) -> (-290, -640)
  line L45 (-290, -640) -> (-290, -600)
  line L46 (-290, -600) -> (-370, -600)
  line L47 (-370, -600) -> (-370, -640)
  dimension "d151" = 80
  dimension "d152" = 40
  constraint horizontal L44
  constraint vertical L45
  constraint horizontal L46
  constraint vertical L47
  measures "d151" distance of L44.start L44.end
  measures "d152" distance of L44.start L46.end
extrude "Extrude24" cut sketch "Sketch49" against normal blind 3 contours L44 L45 L46 L47 bodies 7
sketch "Sketch50" plane through (375.0128, 0, 0) normal (1, 0, 0) x (0, 1, 0)
  circle A0 centre (-209.4172, 16.3577) radius 7.5
  line L0 (-406, 50) -> (-406, 0)
  line L1 (-406, 0) -> (-106, 0)
  line L2 (-106, 0) -> (-106, 50)
  line L3 (-106, 50) -> (-109, 50)
  line L4 (-109, 50) -> (-109, 53)
  line L5 (-109, 53) -> (-209, 53)
  line L6 (-209, 53) -> (-209, 50)
  line L7 (-209, 50) -> (-303, 50)
  line L8 (-303, 50) -> (-303, 53)
  line L9 (-303, 53) -> (-403, 53)
  line L10 (-403, 53) -> (-403, 50)
  line L11 (-403, 50) -> (-406, 50)
  line L12 (-225, 23) -> (-239, 23)
  line L13 (-239, 23) -> (-239, 9)
  line L14 (-239, 9) -> (-225, 9)
  line L15 (-225, 9) -> (-225, 23)
  dimension "d155" = 14
  dimension "d156" = 14
  constraint horizontal L12
  constraint vertical L13
  constraint horizontal L14
  constraint vertical L15
  measures "d155" distance of L12.start L12.end
  measures "d156" distance of L12.start L14.end
extrude "Extrude25" cut sketch "Sketch50" against normal blind 3 contours L12 L13 L14 L15 bodies 4
sketch "Base" plane through (0, 0, 0) normal (0, 0, 1) x (-1, 0, 0)
  line L0 (22, 209) -> (25, 209)
  line L1 (25, 209) -> (25, 303)
  line L2 (25, 303) -> (22, 303)
  line L3 (22, 303) -> (22, 403)
  line L4 (22, 403) -> (25, 403)
  line L5 (25, 403) -> (25, 406)
  line L6 (25, 406) -> (-1.5, 406)
  line L7 (-1.5, 406) -> (-1.5, 403)
  line L8 (-1.5, 403) -> (-101.5, 403)
  line L9 (-101.5, 403) -> (-101.5, 406)
  line L10 (-101.5, 406) -> (-125, 406)
  line L11 (-125, 406) -> (-125, 403)
  line L12 (-125, 403) -> (-225, 403)
  line L13 (-225, 403) -> (-225, 406)
  line L14 (-225, 406) -> (-248.5, 406)
  line L15 (-248.5, 406) -> (-248.5, 403)
  line L16 (-248.5, 403) -> (-348.5, 403)
  line L17 (-348.5, 403) -> (-348.5, 406)
  line L18 (-348.5, 406) -> (-375, 406)
  line L19 (-375, 406) -> (-375, 403)
  line L20 (-375, 403) -> (-372, 403)
  line L21 (-372, 403) -> (-372, 303)
  line L22 (-372, 303) -> (-375, 303)
  line L23 (-375, 303) -> (-375, 209)
  line L24 (-375, 209) -> (-372, 209)
  line L25 (-372, 209) -> (-372, 109)
  line L26 (-372, 109) -> (-375, 109)
  line L27 (-375, 109) -> (-375, 106)
  line L28 (-375, 106) -> (-348.5, 106)
  line L29 (-348.5, 106) -> (-348.5, 109)
  line L30 (-348.5, 109) -> (-248.5, 109)
  line L31 (-248.5, 109) -> (-248.5, 106)
  line L32 (-248.5, 106) -> (-225, 106)
  line L33 (-225, 106) -> (-225, 109)
  line L34 (-225, 109) -> (-125, 109)
  line L35 (-125, 109) -> (-125, 106)
  line L36 (-125, 106) -> (-101.5, 106)
  line L37 (-101.5, 106) -> (-101.5, 109)
  line L38 (-101.5, 109) -> (-1.5, 109)
  line L39 (-1.5, 109) -> (-1.5, 106)
  line L40 (-1.5, 106) -> (25, 106)
  line L41 (25, 106) -> (25, 109)
  line L42 (25, 109) -> (22, 109)
  line L43 (22, 109) -> (22, 209)
sketch "Sketch57" plane through (0, 0, 3) normal (0, 0, 1) x (-1, 0, 0)
  line L0 (-193.5157, -537) -> (-208.5157, -537)
  line L1 (-208.5157, -537) -> (-208.5157, -525)
  line L2 (-208.5157, -525) -> (-193.5157, -525)
  line L3 (-193.5157, -525) -> (-193.5157, -537)
  dimension "d165" = 15
  dimension "d166" = 12
  constraint horizontal L0
  constraint vertical L1
  constraint horizontal L2
  constraint vertical L3
  measures "d165" distance of L0.start L0.end
  measures "d166" distance of L0.start L2.end
extrude "Extrude27" cut sketch "Sketch57" against normal blind 3 bodies 7
sketch "New top" plane through (193.5157, 0, 0) normal (1, 0, 0) x (0, 1, 0)
  line L0 (537, 3) -> (525, 3)
  line L1 (525, 3) -> (525, 0)
  line L2 (525, 0) -> (537, 0)
  line L3 (537, 0) -> (537, 3)
sketch "Sketch60" plane through (0, 0, 3) normal (0, 0, 1) x (-1, 0, 0)
  line L0 (-208.5157, -537) -> (-208.5157, -525)
  line L1 (-208.5157, -525) -> (-193.5157, -525)
  line L2 (-193.5157, -525) -> (-193.5157, -537)
  line L3 (-193.5157, -537) -> (-208.5157, -537)
  line L4 (-290, -640) -> (-370, -640)
  line L5 (-370, -640) -> (-370, -600)
  line L6 (-370, -600) -> (-290, -600)
  line L7 (-290, -600) -> (-290, -640)
  line L8 (-3, -572) -> (0, -572)
  line L9 (0, -572) -> (0, -478)
  line L10 (0, -478) -> (-3, -478)
  line L11 (-3, -478) -> (-3, -378)
  line L12 (-3, -378) -> (0, -378)
  line L13 (0, -378) -> (0, -375)
  line L14 (0, -375) -> (-26.5, -375)
  line L15 (-26.5, -375) -> (-26.5, -378)
  line L16 (-26.5, -378) -> (-126.5, -378)
  line L17 (-126.5, -378) -> (-126.5, -375)
  line L18 (-126.5, -375) -> (-150, -375)
  line L19 (-150, -375) -> (-150, -378)
  line L20 (-150, -378) -> (-250, -378)
  line L21 (-250, -378) -> (-250, -375)
  line L22 (-250, -375) -> (-273.5, -375)
  line L23 (-273.5, -375) -> (-273.5, -378)
  line L24 (-273.5, -378) -> (-373.5, -378)
  line L25 (-373.5, -378) -> (-373.5, -375)
  line L26 (-373.5, -375) -> (-400, -375)
  line L27 (-400, -375) -> (-400, -378)
  line L28 (-400, -378) -> (-397, -378)
  line L29 (-397, -378) -> (-397, -478)
  line L30 (-397, -478) -> (-400, -478)
  line L31 (-400, -478) -> (-400, -572)
  line L32 (-400, -572) -> (-397, -572)
  line L33 (-397, -572) -> (-397, -672)
  line L34 (-397, -672) -> (-400, -672)
  line L35 (-400, -672) -> (-400, -675)
  line L36 (-400, -675) -> (-373.5, -675)
  line L37 (-373.5, -675) -> (-373.5, -672)
  line L38 (-373.5, -672) -> (-273.5, -672)
  line L39 (-273.5, -672) -> (-273.5, -675)
  line L40 (-273.5, -675) -> (-250, -675)
  line L41 (-250, -675) -> (-250, -672)
  line L42 (-250, -672) -> (-150, -672)
  line L43 (-150, -672) -> (-150, -675)
  line L44 (-150, -675) -> (-126.5, -675)
  line L45 (-126.5, -675) -> (-126.5, -672)
  line L46 (-126.5, -672) -> (-26.5, -672)
  line L47 (-26.5, -672) -> (-26.5, -675)
  line L48 (-26.5, -675) -> (0, -675)
  line L49 (0, -675) -> (0, -672)
  line L50 (0, -672) -> (-3, -672)
  line L51 (-3, -672) -> (-3, -572)
sketch "Sketch53" plane through (0, 0, 3) normal (0, 0, 1) x (1, 0, 0)
sketch "Sketch54" plane through (0, 0, 3) normal (0, 0, 1) x (-1, 0, 0)
  line L0 (0, -572) -> (0, -478)
  line L1 (-400, -478) -> (-400, -572)
  line L2 (-250, -672) -> (-150, -672)
  line L3 (-150, -378) -> (-250, -378)
extrude "Extrude26" [suppressed]
sketch "Sketch11" plane through (0, 0, 0) normal (0, 0, -1) x (1, 0, 0)
  line L0 (397, -3) -> (397, 0)
  line L1 (397, 0) -> (3, 0)
  line L2 (3, 0) -> (3, -3)
  line L3 (3, -3) -> (397, -3)
  line L4 (3, 0) -> (50, 0)
  line L5 (50, 0) -> (50, -3)
  line L6 (3, -3) -> (3, 0)
  dimension "d26" = 47
  constraint horizontal L4
  constraint vertical L5
  constraint vertical L6
  constraint coincident L1.end L2.start
  measures "d26" distance of L1.end L4.end
sketch "Sketch12" plane through (0, 0, 0) normal (0, 0, -1) x (1, 0, 0)
  line L0 (50, 0) -> (150, 0)
  line L1 (150, 0) -> (150, -2.8951)
  line L2 (150, -2.8951) -> (50, -2.8951)
  line L3 (50, -2.8951) -> (50, 0)
  dimension "d27" = 100
  constraint horizontal L0
  constraint vertical L1
  constraint horizontal L2
  constraint vertical L3
  measures "d27" distance of L0.start L0.end
